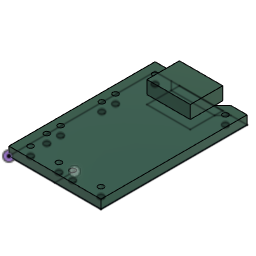
TP4056 Battery Charger v4 (Autodesk Fusion 360 design; units mm, degrees)
Autodesk Fusion 360 part; units mm, degrees
sketch "Skizze1" plane through (0, 0, 0) normal (0, 0, 1) x (1, 0, 0)
  line L0 (0, 0) -> (17, 0)
  line L1 (17, 0) -> (17, 27)
  line L2 (17, 27) -> (0, 27)
  line L3 (0, 27) -> (0, 0)
  line L4 (14, 27) -> (12.5, 25.5)
  line L5 (12.5, 25.5) -> (4.5, 25.5)
  line L6 (4.5, 25.5) -> (3, 27)
  line L7 (4.5, 27) -> (12.5, 27)
  line L8 (12.5, 27) -> (12.5, 21)
  line L9 (12.5, 21) -> (4.5, 21)
  line L10 (4.5, 21) -> (4.5, 27)
  circle A0 centre (2, 25) radius 0.5
  circle A1 centre (15, 25) radius 0.5
  circle A2 centre (2, 2) radius 0.5
  circle A3 centre (15, 2) radius 0.5
  circle A4 centre (7.23, 2) radius 0.5
  circle A5 centre (9.77, 2) radius 0.5
  line L11 (8.5, 0) -> (8.5, 3.6203)
  circle A6 centre (1.5, 5.5) radius 0.5
  circle A7 centre (1.5, 8.04) radius 0.5
  circle A8 centre (1.5, 15.66) radius 0.5
  circle A9 centre (1.5, 18.2) radius 0.5
  dimension "d1" = 17
  dimension "d2" = 27
  dimension "d3" = 3
  dimension "d4" = 3
  dimension "d5" = 45
  dimension "d6" = 45
  dimension "d7" = 1.5
  dimension "d8" = 8
  dimension "d9" = 6
  dimension "d10" = 4.5
  dimension "d17" = 1
  dimension "d18" = 2
  dimension "d19" = 2
  dimension "d22" = 13
  dimension "d23" = -23
  dimension "d24" = 1
  dimension "d25" = 2
  dimension "d28" = 2.54
  dimension "d29" = 0
  dimension "d30" = 1
  dimension "d31" = 5.5
  dimension "d32" = 1.5
  dimension "d35" = 0
  dimension "d36" = 2.54
  dimension "d39" = 0
  dimension "d40" = 10.16
  constraint horizontal L0
  constraint vertical L1
  constraint horizontal L2
  constraint vertical L3
  constraint coincident L0.start L3.end
  constraint coincident L2 L4.start
  constraint perpendicular L1 L5
  constraint coincident L2 L6.end
  constraint horizontal L7
  constraint vertical L8
  constraint horizontal L9
  constraint vertical L10
  constraint collinear L2 L7
  constraint midpoint L0 L11.start
  constraint perpendicular L0 L11
  constraint symmetric A4 A5 L11
  measures "d1" distance of L0.start L0.end
  measures "d2" distance of L0.start L2.end
  measures "d3" distance of L2.end L6.end
  measures "d4" distance of L1.end L4.start
  measures "d5" angle of L2 L4
  measures "d6" angle of L2 L6
  measures "d7" distance of L2 L5
  measures "d8" distance of L7.start L7.end
  measures "d9" distance of L7.start L9.end
  measures "d10" distance of L3 L10
  measures "d17" diameter of A0
  measures "d18" distance of L3 A0.centre
  measures "d19" distance of L2 A0.centre
  measures "d24" diameter of A4
  measures "d25" distance of L0 A4.centre
  measures "d30" diameter of A6
  measures "d31" distance of L0 A6.centre
  measures "d32" distance of L3 A6.centre
extrude "Extrusion2" add sketch "Skizze1" along normal blind 4 contours L2 L5 L7 L8 L10 | L5 L8 L9 L10
extrude "Extrusion3" cut sketch "Skizze1" along normal blind 1.6 contours L2 L5 L7 L8 L10
extrude "Extrusion4" add sketch "Skizze1" along normal blind 1.6 contours L0 L1 L2 L3 L4 L6 L8 L9 L10
sketch "Skizze2" plane through (0, 0, 1.6) normal (0, 0, 1) x (-1, 0, 0)
  circle A0 centre (-1.5, -15.66) radius 0.5
  circle A1 centre (-2, -2) radius 0.5
  circle A2 centre (-1.5, -8.04) radius 0.5
  circle A3 centre (-15, -25) radius 0.5
  circle A4 centre (-1.5, -18.2) radius 0.5
  circle A5 centre (-7.23, -2) radius 0.5
  circle A6 centre (-1.5, -5.5) radius 0.5
  circle A7 centre (-15, -2) radius 0.5
  circle A8 centre (-9.77, -2) radius 0.5
  circle A9 centre (-2, -25) radius 0.5
  line L0 (-4.5, -21) -> (-4.5, -25.5)
  line L1 (-4.5, -25.5) -> (-3, -27)
  line L2 (-3, -27) -> (0, -27)
  line L3 (0, -27) -> (0, 0)
  line L4 (0, 0) -> (-17, 0)
  line L5 (-17, 0) -> (-17, -27)
  line L6 (-17, -27) -> (-14, -27)
  line L7 (-14, -27) -> (-12.5, -25.5)
  line L8 (-12.5, -25.5) -> (-12.5, -21)
  line L9 (-12.5, -21) -> (-4.5, -21)
  line L10 (-4.75, -3.5) -> (-12.25, -3.5)
  line L11 (-12.25, -3.5) -> (-12.25, 7.5)
  line L12 (-12.25, 7.5) -> (-4.75, 7.5)
  line L13 (-4.75, 7.5) -> (-4.75, -3.5)
  line L14 (-4.75, 0) -> (-12.25, 0)
  line L15 (0, 0) -> (-17, 0)
  dimension "d43" = 7.5
  dimension "d44" = 11
  dimension "d45" = 3.5
  constraint horizontal L10
  constraint vertical L11
  constraint horizontal L12
  constraint vertical L13
  constraint coincident L13 L14.start
  constraint coincident L11 L14.end
  constraint perpendicular L11 L14
  constraint midpoint L14 L15
  measures "d43" distance of L10.start L10.end
  measures "d44" distance of L10.start L12.end
  measures "d45" distance of L10 L14
extrude "Extrusion5" [suppressed]
